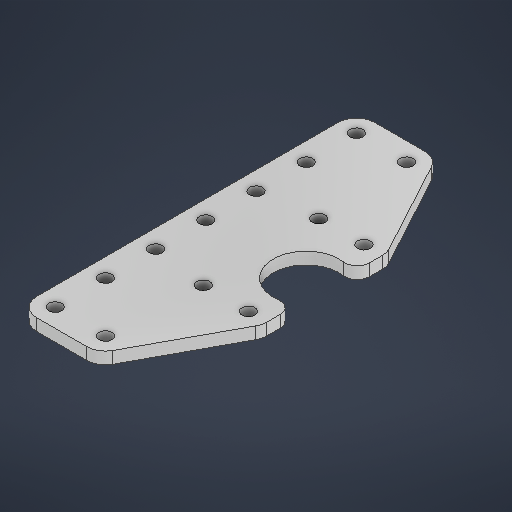
# Autodesk Inventor part: CNC-007-XAxisBallScrewMount
Saved by Autodesk Inventor 2026.2 (Build 302298000, 298)
## iProperties
Created: 2026-06-15
Part Number: CNC-007-XAxisBallScrewMount
Material: Aluminum 6061
Document SubType Name: Modeling
Designer: Kenji
Density: 2.7 g/cm^3
Appearance: Aluminum - Dark
Author: Kenji
Autodesk Inventor part; units mm, degrees
ref_plane "YZ Plane" through (0, 0, 0) normal (1, 0, 0) x (0, 1, 0)
ref_plane "XZ Plane" through (0, 0, 0) normal (0, 1, 0) x (-1, 0, 0)
ref_plane "XY Plane" through (0, 0, 0) normal (0, 0, 1) x (1, 0, 0)
sketch "Sketch1" plane through (0, 0, 0) normal (0, 1, 0) x (-1, 0, 0)
  circle A0 centre (0, 0) radius 2.6
  line L0 (0, 0) -> (0, -2.6) construction
  line L1 (0, 0) -> (-2.6, 0) construction
  circle A1 centre (0, -20) radius 2.6
  circle A2 centre (0, -40) radius 2.6
  circle A3 centre (0, -60) radius 2.6
  circle A4 centre (0, -80) radius 2.6
  circle A5 centre (0, -100) radius 2.6
  circle A6 centre (0, -120) radius 2.6
  circle A7 centre (-20, 0) radius 2.6
  circle A8 centre (-20, -120) radius 2.6
  circle A9 centre (-22, -37) radius 2.6
  line L2 (-22, -37) -> (-22, -39.6) construction
  line L3 (-22, -37) -> (-24.6, -37) construction
  circle A10 centre (-22, -83) radius 2.6
  circle A11 centre (-40, -37) radius 2.6
  circle A12 centre (-40, -83) radius 2.6
  circle A13 centre (0, 0) radius 7.3625 construction
  circle A14 centre (-20, 0) radius 7.3625 construction
  circle A15 centre (-40, -37) radius 7.3625 construction
  circle A16 centre (-40, -83) radius 7.3625 construction
  circle A17 centre (-20, -120) radius 7.3625 construction
  circle A18 centre (0, -120) radius 7.3625 construction
  circle A19 centre (-40, -60) radius 13.15 construction
  line L4 (7.3625, 0) -> (7.3625, -120)
  line L5 (0, -127.3625) -> (-20, -127.3625)
  line L6 (0, 7.3625) -> (-20, 7.3625)
  line L7 (-26.4768, 3.501) -> (-46.4768, -33.499)
  line L8 (-46.4768, -86.501) -> (-26.4768, -123.501)
  line L9 (-47.3625, -37) -> (-47.3625, -42.2772)
  line L10 (-47.3625, -83) -> (-47.3625, -77.7228)
  arc A20 (-41.9087, -73.0107) -> (-41.9087, -46.9893) centre (-40, -60) ccw
  arc A21 (-47.3625, -42.2772) -> (-41.9087, -46.9893) centre (-42.6, -42.2772) ccw
  arc A22 (-41.9087, -73.0107) -> (-47.3625, -77.7228) centre (-42.6, -77.7228) ccw
  arc A23 (-47.3625, -83) -> (-46.4768, -86.501) centre (-40, -83) ccw
  arc A24 (-46.4768, -33.499) -> (-47.3625, -37) centre (-40, -37) ccw
  arc A25 (-20, 7.3625) -> (-26.4768, 3.501) centre (-20, 0) ccw
  arc A26 (7.3625, 0) -> (0, 7.3625) centre (0, 0) ccw
  arc A27 (0, -127.3625) -> (7.3625, -120) centre (0, -120) ccw
  arc A28 (-26.4768, -123.501) -> (-20, -127.3625) centre (-20, -120) ccw
  point P0 (0, -22.6)
  point P1 (-2.6, -20)
  point P2 (0, -42.6)
  point P3 (-2.6, -40)
  point P4 (0, -62.6)
  point P5 (-2.6, -60)
  point P6 (0, -82.6)
  point P7 (-2.6, -80)
  point P8 (0, -102.6)
  point P9 (-2.6, -100)
  point P10 (0, -122.6)
  point P11 (-2.6, -120)
  point P12 (-22, -85.6)
  point P13 (-24.6, -83)
  point P14 (-40, -39.6)
  point P15 (-42.6, -37)
  point P16 (-40, -85.6)
  point P17 (-42.6, -83)
  point P18 (-47.3625, -49.1043)
  point P19 (-47.3625, -70.8957)
  dimension "d0" = 5.2
  dimension "d3" = 20
  dimension "d8" = 20
  dimension "d9" = 37
  dimension "d10" = 2
  dimension "d13" = 46
  dimension "d16" = 18
  dimension "d19" = 4.7625
  dimension "d20" = 26.3
  dimension "d21" = 23
  dimension "d22" = 4.7625
  constraints: 56 point on circle, 29 centre point, 22 end point, 17 tangent, 14 equal radius, 6 coincident, 6 vertical, 3 horizontal, 2 horizontal alignment, 2 perpendicular, 2 point on line, 2 vertical alignment, 1 concentric, 36 other
  measures "d0" diameter of A0
  measures "d3" distance of L0.start A1.centre
  measures "d8" distance of A7.centre point (0, 0)
  measures "d9" vertical distance of A7.centre L2.start
  measures "d10" horizontal distance of L2.start A7.centre
  measures "d13" distance of L2.start A10.centre
  measures "d16" distance of L2.start A11.centre
  measures "d19" radial gap between concentric circles of A13 A0
  measures "d20" diameter of A19
  measures "d21" distance of A19.centre A11.centre
  measures "d22" radius of A21
extrude "Extrusion1" add sketch "Sketch1" along normal blind 4.7625
body "Solid1"
